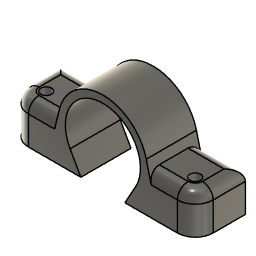
CHASSI_PowerSwitch_HOLDER (Autodesk Fusion 360 design; units mm, degrees)
Autodesk Fusion 360 part; units mm, degrees
sketch "Sketch1" plane through (0, 0, 69) normal (0, 0, 1) x (-1, 0, 0)
  circle A0 centre (29.17, 30.575) radius 3.05
  circle A1 centre (70.83, 30.575) radius 3.05
  line L0 (24.17, 21.15) -> (75.83, 21.15)
  line L1 (75.83, 21.15) -> (75.83, 30.575)
  arc A2 (75.83, 30.575) -> (70.83, 35.575) centre (70.83, 30.575) ccw
  line L2 (70.83, 35.575) -> (29.17, 35.575)
  arc A3 (29.17, 35.575) -> (24.17, 30.575) centre (29.17, 30.575) ccw
  line L3 (24.17, 30.575) -> (24.17, 21.15)
  line L4 (29.8595, -5) -> (27.8595, -5)
  arc A4 (23.8595, -1) -> (27.8595, -5) centre (27.8595, -1) ccw
  line L5 (23.8595, -1) -> (23.8595, 1)
  arc A5 (27.8595, 5) -> (23.8595, 1) centre (27.8595, 1) ccw
  line L6 (27.8595, 5) -> (29.8595, 5)
  arc A6 (33.8595, 1) -> (29.8595, 5) centre (29.8595, 1) ccw
  line L7 (33.8595, 1) -> (33.8595, -1)
  arc A7 (29.8595, -5) -> (33.8595, -1) centre (29.8595, -1) ccw
  circle A8 centre (50, 0) radius 10
  line L8 (76.1405, 1) -> (76.1405, -1)
  arc A9 (72.1405, -5) -> (76.1405, -1) centre (72.1405, -1) ccw
  line L9 (72.1405, -5) -> (70.1405, -5)
  arc A10 (66.1405, -1) -> (70.1405, -5) centre (70.1405, -1) ccw
  line L10 (66.1405, -1) -> (66.1405, 1)
  arc A11 (70.1405, 5) -> (66.1405, 1) centre (70.1405, 1) ccw
  line L11 (70.1405, 5) -> (72.1405, 5)
  arc A12 (76.1405, 1) -> (72.1405, 5) centre (72.1405, 1) ccw
  circle A13 centre (95.6212, 10.575) radius 1.5
  circle A14 centre (37.085, 10.575) radius 1.5
  circle A15 centre (62.915, 10.575) radius 1.5
  circle A16 centre (37.085, -10.575) radius 1.5
  circle A17 centre (62.915, -10.575) radius 1.5
  circle A18 centre (4.3788, 10.575) radius 1.5
  circle A19 centre (95.6212, -10.575) radius 1.5
  circle A20 centre (4.3788, -10.575) radius 1.5
  line L12 (-10, -21.15) -> (110, -21.15)
  line L13 (110, -21.15) -> (110, 21.15)
  line L14 (110, 21.15) -> (-10, 21.15)
  line L15 (-10, 21.15) -> (-10, -21.15)
  line L16 (24.17, 21.55) -> (75.83, 21.55)
  dimension "d176" = -0.4
extrude "Extrude1" add sketch "Sketch1" along normal blind 2 contours L1 A2 L2 A3 L3 L16
sketch "Sketch2" plane through (0, -35.575, 0) normal (0, -1, 0) x (1, 0, 0)
  line L0 (-70.83, 69) -> (-29.17, 69)
  line L1 (-29.17, 69) -> (-29.17, 71)
  line L2 (-29.17, 71) -> (-70.83, 71)
  line L3 (-70.83, 71) -> (-70.83, 69)
  line L4 (9.9999, 77.6216) -> (10, 92) construction
  line L5 (10, 92) -> (-110, 92) construction
  line L6 (-110, 92) -> (-109.9999, 77.6216) construction
  line L7 (-109.9999, 77.6216) -> (-98.6213, 89) construction
  line L8 (-98.6213, 89) -> (-92.6213, 89) construction
  line L9 (-92.6213, 89) -> (-81.2425, 77.621) construction
  line L10 (-81.2425, 77.621) -> (-81.2425, 89) construction
  line L11 (-81.2425, 89) -> (-18.7575, 89) construction
  line L12 (-18.7575, 89) -> (-18.7575, 77.621) construction
  line L13 (-18.7575, 77.621) -> (-7.3788, 89) construction
  line L14 (-7.3788, 89) -> (-1.3788, 89) construction
  line L15 (-1.3788, 89) -> (9.9999, 77.6216) construction
  line L16 (-50, 70) -> (-50, 89)
  circle A0 centre (-50, 79.5) radius 10.5
  arc A1 (-40.8349, 71) -> (-59.1652, 71) centre (-50, 79.5) ccw
  line L17 (-59.1652, 71) -> (-70.83, 71) construction
  line L18 (-40.8349, 71) -> (-29.17, 71) construction
  line L19 (-64.9976, 71) -> (-62.1298, 82.5197)
  line L20 (-35.0024, 71) -> (-37.8702, 82.5197)
  dimension "d179" = 21
  constraint midpoint L11 L16.end
  constraint midpoint L16 A0.centre
  constraint concentric A0 A1
  constraint coincident L2 A1.end
  constraint coincident L2 A1.start
  constraint coincident L2.end L3.start
  constraint coincident L1.end L2.start
  constraint midpoint L17 L19.start
  constraint coincident A1 L19.end
  constraint tangent A1 L19
  constraint midpoint L18 L20.start
  constraint coincident A1 L20.end
  constraint tangent A1 L20
  measures "d179" diameter of A0
extrude "Extrude2" add sketch "Sketch2" against normal blind 14.025 contours L2 A0 A1 | L2 A1 L19 | L2 A1 L20
sketch "Sketch3" plane through (0, -35.575, 0) normal (0, -1, 0) x (1, 0, 0)
  line L0 (-64.9976, 71) -> (-70.83, 71)
  line L1 (-70.83, 71) -> (-70.83, 69)
  line L2 (-70.83, 69) -> (-29.17, 69)
  line L3 (-29.17, 69) -> (-29.17, 71)
  line L4 (-29.17, 71) -> (-35.0024, 71)
  line L5 (-35.0024, 71) -> (-37.8702, 82.5197)
  arc A0 (-37.8702, 82.5197) -> (-62.1298, 82.5197) centre (-50, 79.5) ccw
  line L6 (-62.1298, 82.5197) -> (-64.9976, 71)
  arc A1 (-43.8356, 71) -> (-56.1644, 71) centre (-50, 79.5) ccw
  line L7 (-43.8356, 71) -> (-56.1644, 71)
  line L8 (-59.1687, 74.3828) -> (-56.1644, 69)
  line L9 (-50, 69) -> (-50, 90) construction
  line L10 (-40.8313, 74.3828) -> (-43.8356, 69)
  arc A2 (-40.8313, 74.3828) -> (-59.1687, 74.3828) centre (-50, 79.5) ccw
  dimension "d183" = 21
  constraint concentric A0 A2
  constraint coincident L2 L8.end
  constraint tangent L8 A2
  constraint midpoint L2 L9.start
  constraint midpoint A1 L9.end
  constraint symmetric L8.end L9 L10.end
  constraint symmetric L8.start L9 L10.start
  measures "d183" diameter of A2
extrude "Extrude3" cut sketch "Sketch3" against normal blind 14.025 contours L2 A1 L7 L8 L10
sketch "Sketch4" plane through (0, 0, 71) normal (0, 0, 1) x (-1, 0, 0)
  line L0 (64.9976, 35.575) -> (64.9976, 21.55)
  line L1 (64.9976, 21.55) -> (75.83, 21.55)
  line L2 (75.83, 21.55) -> (75.83, 30.575)
  arc A0 (75.83, 30.575) -> (70.83, 35.575) centre (70.83, 30.575) ccw
  line L3 (70.83, 35.575) -> (64.9976, 35.575)
  circle A1 centre (70.83, 30.575) radius 3.05
  line L4 (62.1298, 35.575) -> (37.8702, 35.575)
  line L5 (37.8702, 35.575) -> (37.8702, 21.55)
  line L6 (37.8702, 21.55) -> (62.1298, 21.55)
  line L7 (62.1298, 21.55) -> (62.1298, 35.575)
  line L8 (64.9976, 35.575) -> (62.1298, 35.575)
  line L9 (62.1298, 35.575) -> (62.1298, 21.55)
  line L10 (62.1298, 21.55) -> (64.9976, 21.55)
  line L11 (64.9976, 21.55) -> (64.9976, 35.575)
  line L12 (37.8702, 35.575) -> (35.0024, 35.575)
  line L13 (35.0024, 35.575) -> (35.0024, 21.55)
  line L14 (35.0024, 21.55) -> (37.8702, 21.55)
  line L15 (37.8702, 21.55) -> (37.8702, 35.575)
  circle A2 centre (29.17, 30.575) radius 3.05
  line L16 (35.0024, 21.55) -> (35.0024, 35.575)
  line L17 (35.0024, 35.575) -> (29.17, 35.575)
  arc A3 (29.17, 35.575) -> (24.17, 30.575) centre (29.17, 30.575) ccw
  line L18 (24.17, 30.575) -> (24.17, 21.55)
  line L19 (24.17, 21.55) -> (35.0024, 21.55)
  line L20 (50, 21.55) -> (50, 35.575) construction
  circle A4 centre (70.83, 30.575) radius 1.5
  circle A5 centre (29.17, 30.575) radius 1.5
  dimension "d186" = 3
  dimension "d187" = 3
  constraint midpoint L6 L20.start
  constraint midpoint L4 L20.end
  constraint concentric A0 A4
  constraint concentric A2 A5
  measures "d186" diameter of A4
  measures "d187" diameter of A5
extrude "Extrude4" add sketch "Sketch4" against normal blind 2 contours A1 | A2
delete_face "DeleteFace1" 1 faces at (-75.1601, -33.075, 70.3333)
delete_face "DeleteFace2" 1 faces at (-24.445, -32.2103, 70.3333)
sketch "Sketch5" plane through (0, -35.575, 0) normal (0, -1, 0) x (1, 0, 0)
  line L0 (-24.17, 71) -> (-35.0024, 71)
  line L1 (-35.0024, 71) -> (-37.8702, 82.5197)
  arc A0 (-37.8702, 82.5197) -> (-62.1298, 82.5197) centre (-50, 79.5) ccw
  line L2 (-62.1298, 82.5197) -> (-64.9976, 71)
  line L3 (-64.9976, 71) -> (-75.83, 71)
  line L4 (-75.83, 71) -> (-75.83, 69)
  line L5 (-75.83, 69) -> (-56.1644, 69)
  line L6 (-56.1644, 69) -> (-59.1687, 74.3828)
  arc A1 (-40.8313, 74.3828) -> (-59.1687, 74.3828) centre (-50, 79.5) ccw
  line L7 (-40.8313, 74.3828) -> (-43.8356, 69)
  line L8 (-43.8356, 69) -> (-24.17, 69)
  line L9 (-24.17, 69) -> (-24.17, 71)
  line L10 (-70.4138, 71) -> (-70.4138, 80) construction
  line L11 (-50, 92) -> (-50, 68.7831) construction
  line L12 (-75.83, 71) -> (-75.83, 80)
  line L13 (-75.83, 80) -> (-62.7571, 80)
  line L14 (-24.17, 71) -> (-24.17, 80)
  line L15 (-24.17, 80) -> (-37.243, 80)
  dimension "d297" = 9
  constraint midpoint L3 L10.start
  constraint perpendicular L3 L10
  constraint midpoint A0 L11.start
  constraint vertical L11
  constraint coincident L3.end L4.start
  constraint perpendicular L3 L12
  constraint coincident L2 L13.end
  constraint perpendicular L12 L13
  constraint symmetric L11 L3.end L0.start
  constraint symmetric L11 L12.end L14.end
  constraint symmetric L11 L13.end L15.end
  measures "d297" distance of L10.start L10.end
extrude "Extrude5" add sketch "Sketch5" against normal blind 14.025 contours L0 L1 L14 L15 | L2 L3 L12 L13
extrude "Extrude6" cut 2 faces at (-70.0515, -30.2933, 71) (-28.7569, -30.8567, 71) along direction (0, 0, 1) blind 9
fillet "Fillet1" radius 5 5 edges at (-75.83, -35.575, 74.5) (-24.17, -35.575, 75.5) (-24.17, -35.575, 70) (-24.17, -35.575, 75.5) (-24.17, -35.575, 70)
fillet "Fillet2" radius 3 8 edges at (-69.2935, -21.55, 80) (-66.7935, -35.575, 80) (-74.3655, -34.1105, 80) (-75.83, -26.0625, 80) (-30.7065, -21.55, 80) (-33.2065, -35.575, 80) (-25.6345, -34.1105, 80) (-24.17, -26.0625, 80)
